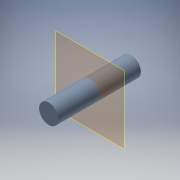
# Autodesk Inventor part: ear
Saved by Autodesk Inventor 2019 (Build 230136000, 136)
## iProperties
Created: 2018-05-20
Part Number: ear
Material: 一般
Document SubType Name: Modeling
Designer: uctom
Density: 1 g/cm^3
Appearance: 淡い鋼色
Author: uctom
Autodesk Inventor part; units mm, degrees
ref_plane "YZ Plane" through (0, 0, 0) normal (1, 0, 0) x (0, 1, 0)
ref_plane "XZ Plane" through (0, 0, 0) normal (0, 1, 0) x (-1, 0, 0)
ref_plane "XY Plane" through (0, 0, 0) normal (0, 0, 1) x (1, 0, 0)
ref_plane "作業平面1" through (0, 0, 0) normal (0, 0, 1) x (1, 0, 0)
sketch "スケッチ2" plane through (0, 0, 0) normal (0, 0, 1) x (1, 0, 0)
  circle A0 centre (0, 15) radius 5 projected
  circle A1 centre (0, 15) radius 4.7
  point P0 (0, 0)
  dimension "d3" = 0.3
  constraints: 1 centre point
  measures "d3" radial gap between concentric circles of A0 A1
extrude "押し出し2" add sketch "スケッチ2" along normal mid plane 40 contours A1
